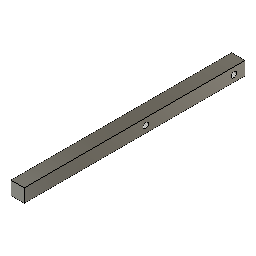
module (Autodesk Fusion 360 archive; units mm, degrees)
design "module_bolt"
Autodesk Fusion 360 part; units mm, degrees
sketch "Skizze1" plane through (0, 0, 0) normal (0, 1, 0) x (1, 0, 0)
  line L0 (0, 0) -> (6, 0)
  line L1 (6, 0) -> (6, -6)
  line L2 (6, -6) -> (0, -6)
  line L3 (0, -6) -> (0, 0)
  dimension "d1" = 6
  dimension "d2" = 6
  constraint horizontal L0
  constraint vertical L1
  constraint horizontal L2
  constraint vertical L3
  constraint coincident L0.start L3.end
  measures "d1" distance of L0.start L0.end
  measures "d2" distance of L0.end L1.end
extrude "Extrusion1" add sketch "Skizze1" along normal blind 100
sketch "Skizze2" plane through (6, 0, 0) normal (1, 0, 0) x (0, 1, 0)
  line L0 (0, 6) -> (0, 0)
  line L1 (0, 0) -> (100, 0)
  line L2 (100, 0) -> (100, 6)
  line L3 (100, 6) -> (0, 6)
  point P0 (95, 3)
  point P1 (55, 3)
  dimension "d5" = 3
  dimension "d6" = 3
  dimension "d7" = 5
  dimension "d8" = 45
  measures "d5" distance of L1 P1
  measures "d6" distance of L1 P0
  measures "d7" distance of L2 P0
  measures "d8" distance of L2 P1
hole "Bohrung1" at (6, 95, 3) at (6, 55, 3) direction (-1, 0, 0) diameter 2.529 depth 30 tip angle 118
thread "Gewinde1" "ISO Metric profile 3.0 M3x0.5 6H"

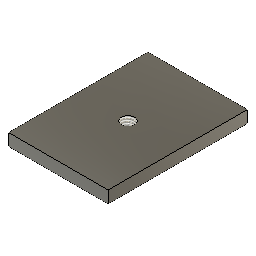
design "module_plate"
Autodesk Fusion 360 part; units mm, degrees
sketch "Skizze1" plane through (0, 0, 0) normal (0, 0, 1) x (1, 0, 0)
  line L0 (-12.5, -17.5) -> (12.5, -17.5)
  line L1 (12.5, -17.5) -> (12.5, 17.5)
  line L2 (12.5, 17.5) -> (-12.5, 17.5)
  line L3 (-12.5, 17.5) -> (-12.5, -17.5)
  dimension "d1" = 25
  dimension "d2" = 35
  dimension "d3" = 17.5
  dimension "d4" = 12.5
  constraint horizontal L0
  constraint vertical L1
  constraint horizontal L2
  constraint vertical L3
  measures "d1" distance of L0.start L0.end
  measures "d2" distance of L0.end L1.end
  measures "d3" distance of origin L2
  measures "d4" distance of origin L3
extrude "Extrusion1" add sketch "Skizze1" along normal blind 3
sketch "Skizze2" plane through (0, 0, 3) normal (0, 0, 1) x (-1, 0, 0)
  line L0 (12.5, -17.5) -> (12.5, 17.5)
  line L1 (12.5, 17.5) -> (-12.5, 17.5)
  line L2 (-12.5, 17.5) -> (-12.5, -17.5)
  line L3 (-12.5, -17.5) -> (12.5, -17.5)
hole "Bohrung1" at (0, 0, 3) direction (0, 0, -1) diameter 3.332 end through all
thread "Gewinde1" "ISO Metric profile 4.0 M4x0.7 6H"
equation "d3 = ( 35 / 2 ) * 1 mm"
equation "d4 = ( 25 / 2 ) * 1 mm"

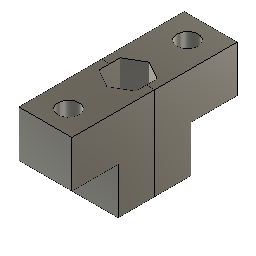
design "module_stand"
Autodesk Fusion 360 part; units mm, degrees
sketch "Skizze1" plane through (0, 0, 0) normal (1, 0, 0) x (0, 1, 0)
  line L0 (0, 0) -> (0, 14)
  line L1 (0, 14) -> (12.5, 14)
  line L2 (12.5, 14) -> (12.5, 7)
  line L3 (12.5, 7) -> (5.5, 7)
  line L4 (5.5, 7) -> (5.5, 0)
  line L5 (5.5, 0) -> (0, 0)
  dimension "d1" = 5.5
  dimension "d2" = 7
  dimension "d3" = 14
  dimension "d4" = 12.5
  constraint coincident L0.start L5.end
  constraint vertical L0
  constraint perpendicular L0 L1
  constraint perpendicular L1 L2
  constraint perpendicular L2 L3
  constraint perpendicular L1 L4
  constraint perpendicular L4 L5
  measures "d1" distance of L0.start L4.end
  measures "d2" distance of L3.end L4.end
  measures "d3" distance of L0.start L0.end
  measures "d4" distance of L0.end L1.end
extrude "Extrusion1" add sketch "Skizze1" along normal blind 8 makes body 1
sketch "Skizze2" plane through (0, 0, 14) normal (0, 0, 1) x (-1, 0, 0)
  line L0 (0, -12.5) -> (0, 0)
  line L1 (0, 0) -> (-8, 0)
  line L2 (-8, 0) -> (-8, -12.5)
  line L3 (-8, -12.5) -> (0, -12.5)
  point P0 (-4, 0)
  point P1 (-4, -9)
  dimension "d7" = 4
  dimension "d8" = 4
  dimension "d10" = 3.5
  constraint coincident L1 P0
  measures "d7" distance of L2 P1
  measures "d8" distance of L2 P0
  measures "d10" distance of L3 P1
hole "Bohrung1" at (4, 0, 14) at (4, 9, 14) direction (0, 0, -1) diameter 3.2 end through all bodies 1
sketch "Skizze3" plane through (0, 0, 14) normal (0, 0, 1) x (-1, 0, 0)
  arc A0 (-5.6, 0) -> (-2.4, 0) centre (-4, 0) ccw
  line L0 (-5.6, 0) -> (-8, 0)
  line L1 (-8, 0) -> (-8, -12.5)
  line L2 (-8, -12.5) -> (0, -12.5)
  line L3 (0, -12.5) -> (0, 0)
  line L4 (0, 0) -> (-2.4, 0)
  circle A1 centre (-4, -9) radius 1.6
  line L5 (-1.2, 1.6166) -> (-4, 3.2332)
  line L6 (-4, 3.2332) -> (-6.8, 1.6166)
  line L7 (-6.8, 1.6166) -> (-6.8, -1.6166)
  line L8 (-6.8, -1.6166) -> (-4, -3.2332)
  line L9 (-4, -3.2332) -> (-1.2, -1.6166)
  line L10 (-1.2, -1.6166) -> (-1.2, 1.6166)
  point P0 (-4, 0)
  dimension "d14" = 5.6
  constraint coincident P0 A0.centre
  constraint parallel L1 L7
  measures "d14" distance of L7 L10
extrude "Extrusion2" cut sketch "Skizze3" against normal blind 7 contours A0 L0 L4 L7 L8 L9 L10 bodies 1
sketch "Skizze4" plane through (0, 0, 7) normal (0, 0, -1) x (1, 0, 0)
  circle A0 centre (4, -9) radius 1.6
  line L0 (0, -5.5) -> (0, -12.5)
  line L1 (0, -12.5) -> (8, -12.5)
  line L2 (8, -12.5) -> (8, -5.5)
  line L3 (8, -5.5) -> (0, -5.5)
  line L4 (6.8, -7.3834) -> (4, -5.7668)
  line L5 (4, -5.7668) -> (1.2, -7.3834)
  line L6 (1.2, -7.3834) -> (1.2, -10.6166)
  line L7 (1.2, -10.6166) -> (4, -12.2332)
  line L8 (4, -12.2332) -> (6.8, -10.6166)
  line L9 (6.8, -10.6166) -> (6.8, -7.3834)
  point P0 (4, -9)
  dimension "d17" = 5.6
  constraint coincident P0 A0.centre
  constraint parallel L0 L6
  measures "d17" distance of L6 L9
extrude "Extrusion3" cut sketch "Skizze4" against normal blind 4 contours L4 L5 L6 L7 L8 L9 bodies 1
mirror "Spiegeln1" about plane through (0, 0, 0) normal (0, -1, 0) of "Extrusion1", "Bohrung1", "Extrusion2", "Extrusion3" makes body 2
equation "d1 = ( 11 / 2 ) * 1 mm"
equation "d4 = ( 25 / 2 ) * 1 mm"

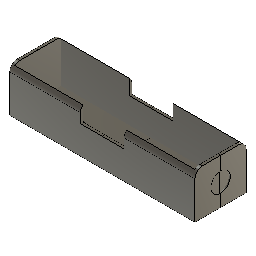
design "18620_holder"
Autodesk Fusion 360 part; units mm, degrees
sketch "Skizze1" plane through (0, 0, 0) normal (0, 0, 1) x (1, 0, 0)
  line L0 (0, 0) -> (38, 0)
  line L1 (38, 0) -> (38, 10.5)
  line L2 (38, 10.5) -> (0, 10.5)
  line L3 (0, 10.5) -> (0, 0)
  dimension "d1" = 38
  dimension "d2" = 10.5
  constraint horizontal L0
  constraint vertical L1
  constraint horizontal L2
  constraint vertical L3
  constraint coincident L0.start L3.end
  measures "d1" distance of L0.start L0.end
  measures "d2" distance of L0.end L1.end
extrude "Extrusion1" add sketch "Skizze1" along normal blind 18.5 makes body 1
shell "Schale1" thickness 1 removed faces 3 at (12.6667, 0, 6.1667) at (0, 3.5, 12.3333) at (25.3333, 3.5, 18.5) on bodies 1
fillet "Abrundung1" radius 3 1 edges at (19, 10.5, 18.5) on bodies 1
sketch "Skizze2" plane through (38, 0, 0) normal (1, 0, 0) x (0, 1, 0)
  arc A0 (10.5, 15.5) -> (7.5, 18.5) centre (7.5, 15.5) ccw
  line L0 (7.5, 18.5) -> (0, 18.5)
  line L1 (0, 18.5) -> (0, 0)
  line L2 (0, 0) -> (10.5, 0)
  line L3 (10.5, 0) -> (10.5, 15.5)
  circle A1 centre (0, 9) radius 4
  dimension "d8" = 9
  dimension "d9" = 8
  constraint coincident L1 A1.centre
  measures "d8" distance of L2 A1.centre
  measures "d9" diameter of A1
extrude "Extrusion2" cut sketch "Skizze2" against normal blind 0.5 contours L1 A1 picked at (1.594, 7.7807) bodies 1
sketch "Skizze3" plane through (0, 0, 18.5) normal (0, 0, 1) x (-1, 0, 0)
  line L0 (-38, -7.5) -> (-37, -7.5)
  line L1 (-37, -7.5) -> (-37, 0)
  line L2 (-37, 0) -> (-38, 0)
  line L3 (-38, 0) -> (-38, -7.5)
  line L4 (0, -9.5) -> (-9, -9.5)
  line L5 (-9, -9.5) -> (-9, -11.5)
  line L6 (-9, -11.5) -> (0, -11.5)
  line L7 (0, -11.5) -> (0, -9.5)
  line L8 (-37, 0) -> (0, 0)
  line L9 (0, 0) -> (0, -9.5)
  dimension "d12" = 9
  dimension "d13" = 2
  dimension "d14" = 9.5
  dimension "d16" = 29
  constraint horizontal L4
  constraint vertical L5
  constraint horizontal L6
  constraint vertical L7
  measures "d12" distance of L4.start L4.end
  measures "d13" distance of L4.end L5.end
  measures "d14" distance of L4 L8
  measures "d16" distance of L3 L5
extrude "Extrusion3" cut sketch "Skizze3" against normal blind 7 contours L4 L5 L6 L7 bodies 1
sketch "Skizze4" plane through (0, 0, 1) normal (0, 0, 1) x (-1, 0, 0)
  line L0 (0, -9.5) -> (0, 0)
  line L1 (0, 0) -> (-37, 0)
  line L2 (-37, 0) -> (-37, -9.5)
  line L3 (-37, -9.5) -> (0, -9.5)
  point P0 (-20, 0)
  dimension "d26" = 20
  constraint coincident L0.end L1.start
  constraint coincident L1 P0
  measures "d26" distance of L0.end P0
hole "Bohrung1" at (0, 0, 1) at (20, 0, 1) direction (0, 0, -1) diameter 3.2 depth 10 tip angle 118 bodies 1
mirror "Spiegeln1" about plane through (0, 0, 0) normal (0, 1, 0) of "Extrusion1", "Schale1", "Abrundung1", "Extrusion2", "Extrusion3", "Bohrung1" makes body 2
mirror "Spiegeln2" about plane through (0, 0, 0) normal (1, 0, 0) of "Extrusion1", "Schale1", "Abrundung1", "Extrusion2", "Extrusion3", "Bohrung1", "Spiegeln1" makes body 3 at (-27.6667, 9.5, 10.0787) makes body 4 at (-27.6667, -9.5, 10.0787)
equation "d1 = ( 76 / 2 ) * 1 mm"
equation "d2 = ( 21 / 2 ) * 1 mm"
equation "d16 = ( 76 / 2 ) * 1 mm - 9 mm"
